Autodesk Inventor part; units mm, degrees
(part 2 of 2)
sketch "스케치10" plane through (0, 0, 4) normal (0, 0, 1) x (1, 0, 0)
  circle A0 centre (0, 0) radius 1.25 projected
  arc A1 (13.9479, -1.2066) -> (10.7334, 8.9886) centre (0, 0) ccw projected
  arc A2 (8.9665, -0.7757) -> (13.9479, -1.2066) centre (11.4572, -0.9911) ccw projected
  arc A3 (8.9665, -0.7757) -> (6.9, 5.7784) centre (0, 0) ccw projected
  arc A4 (10.7334, 8.9886) -> (6.9, 5.7784) centre (8.8167, 7.3835) ccw projected
  arc A5 (-8.0189, -11.476) -> (2.4176, -13.7897) centre (0, 0) ccw projected
  arc A6 (-5.155, -7.3774) -> (-8.0189, -11.476) centre (-6.5869, -9.4267) ccw projected
  arc A7 (-5.155, -7.3774) -> (1.5542, -8.8648) centre (0, 0) ccw projected
  arc A8 (2.4176, -13.7897) -> (1.5542, -8.8648) centre (1.9859, -11.3272) ccw projected
  arc A9 (-3.8115, 8.1531) -> (-8.4542, 3.0864) centre (0, 0) ccw projected
  arc A10 (-13.151, 4.8011) -> (-8.4542, 3.0864) centre (-10.8026, 3.9438) ccw projected
  arc A11 (-5.929, 12.6825) -> (-13.151, 4.8011) centre (0, 0) ccw projected
  arc A12 (-3.8115, 8.1531) -> (-5.929, 12.6825) centre (-4.8703, 10.4178) ccw projected
  circle A13 centre (-59.4867, -7.8316) radius 4.025 projected
  arc A14 (-60.1049, -2.02) -> (-65.4557, -8.4603) centre (-59.4744, -7.9868) ccw projected
  arc A15 (-65.4557, -8.4603) -> (-58.5717, -13.6038) centre (-59.507, -7.6772) ccw projected
  line L0 (-58.5717, -13.6038) -> (-20.5345, -7.6012) projected
  arc A16 (-19.9916, -7.9111) -> (-20.5345, -7.6012) centre (-20.4565, -8.0951) ccw projected
  arc A17 (-19.9916, -7.9111) -> (-19.7349, -8.5314) centre (0, 0) ccw projected
  arc A18 (-19.9027, -9.1363) -> (-19.7349, -8.5314) centre (-20.1938, -8.7298) ccw projected
  arc A19 (-19.9027, -9.1363) -> (-22.7962, -12.5032) centre (-14.4518, -16.7475) ccw projected
  arc A20 (-22.7962, -12.5032) -> (-22.2262, -13.4905) centre (0, 0) ccw projected
  arc A21 (-22.2262, -13.4905) -> (-17.8636, -12.6681) centre (-21.7297, -4.1418) ccw projected
  arc A22 (-17.2558, -12.8252) -> (-17.8636, -12.6681) centre (-17.6571, -13.1235) ccw projected
  arc A23 (-17.2558, -12.8252) -> (-16.8544, -13.3484) centre (0, 0) ccw projected
  arc A24 (-16.8599, -13.9762) -> (-16.8544, -13.3484) centre (-17.2463, -13.6589) ccw projected
  arc A25 (-16.8599, -13.9762) -> (-18.7834, -17.9773) centre (-9.6248, -19.9173) ccw projected
  arc A26 (-18.7834, -17.9773) -> (-17.9773, -18.7834) centre (0, 0) ccw projected
  arc A27 (-17.9773, -18.7834) -> (-13.9762, -16.8599) centre (-19.9173, -9.6248) ccw projected
  arc A28 (-13.3484, -16.8544) -> (-13.9762, -16.8599) centre (-13.6589, -17.2463) ccw projected
  arc A29 (-13.3484, -16.8544) -> (-12.8252, -17.2558) centre (0, 0) ccw projected
  arc A30 (-12.6681, -17.8636) -> (-12.8252, -17.2558) centre (-13.1235, -17.6571) ccw projected
  arc A31 (-12.6681, -17.8636) -> (-13.4905, -22.2262) centre (-4.1418, -21.7297) ccw projected
  arc A32 (-13.4905, -22.2262) -> (-12.5032, -22.7962) centre (0, 0) ccw projected
  arc A33 (-12.5032, -22.7962) -> (-9.1363, -19.9027) centre (-16.7475, -14.4518) ccw projected
  arc A34 (-8.5314, -19.7349) -> (-9.1363, -19.9027) centre (-8.7298, -20.1938) ccw projected
  arc A35 (-8.5314, -19.7349) -> (-7.9221, -19.9873) centre (0, 0) ccw projected
  arc A36 (-7.613, -20.5337) -> (-7.9221, -19.9873) centre (-8.1063, -20.4521) ccw projected
  arc A37 (-7.613, -20.5337) -> (-7.2783, -24.9605) centre (1.6233, -22.0613) ccw projected
  arc A38 (-7.2783, -24.9605) -> (-6.1771, -25.2556) centre (0, 0) ccw projected
  arc A39 (-6.1771, -25.2556) -> (-3.6738, -21.5892) centre (-12.4365, -18.2939) ccw projected
  arc A40 (-3.1329, -21.2705) -> (-3.6738, -21.5892) centre (-3.2058, -21.7652) ccw projected
  arc A41 (-3.1329, -21.2705) -> (-2.4791, -21.3566) centre (0, 0) ccw projected
  arc A42 (-2.0391, -21.8044) -> (-2.4791, -21.3566) centre (-2.5367, -21.8533) ccw projected
  arc A43 (-2.0391, -21.8044) -> (-0.57, -25.9938) centre (7.2779, -20.8894) ccw projected
  arc A44 (-0.57, -25.9938) -> (0.57, -25.9938) centre (0, 0) ccw projected
  arc A45 (0.57, -25.9938) -> (2.0391, -21.8044) centre (-7.2779, -20.8894) ccw projected
  arc A46 (2.4791, -21.3566) -> (2.0391, -21.8044) centre (2.5367, -21.8533) ccw projected
  arc A47 (2.4791, -21.3566) -> (3.1329, -21.2705) centre (0, 0) ccw projected
  arc A48 (3.6738, -21.5892) -> (3.1329, -21.2705) centre (3.2058, -21.7652) ccw projected
  arc A49 (3.6738, -21.5892) -> (6.1771, -25.2556) centre (12.4365, -18.2939) ccw projected
  arc A50 (6.1771, -25.2556) -> (7.2783, -24.9605) centre (0, 0) ccw projected
  arc A51 (7.2783, -24.9605) -> (7.613, -20.5337) centre (-1.6233, -22.0613) ccw projected
  arc A52 (7.9221, -19.9873) -> (7.613, -20.5337) centre (8.1063, -20.4521) ccw projected
  arc A53 (7.9221, -19.9873) -> (8.5314, -19.7349) centre (0, 0) ccw projected
  arc A54 (9.1363, -19.9027) -> (8.5314, -19.7349) centre (8.7298, -20.1938) ccw projected
  arc A55 (9.1363, -19.9027) -> (12.5032, -22.7962) centre (16.7475, -14.4518) ccw projected
  arc A56 (12.5032, -22.7962) -> (13.4905, -22.2262) centre (0, 0) ccw projected
  arc A57 (13.4905, -22.2262) -> (12.6681, -17.8636) centre (4.1418, -21.7297) ccw projected
  arc A58 (12.8252, -17.2558) -> (12.6681, -17.8636) centre (13.1235, -17.6571) ccw projected
  arc A59 (12.8252, -17.2558) -> (13.3484, -16.8544) centre (0, 0) ccw projected
  arc A60 (13.9762, -16.8599) -> (13.3484, -16.8544) centre (13.6589, -17.2463) ccw projected
  arc A61 (13.9762, -16.8599) -> (17.9773, -18.7834) centre (19.9173, -9.6248) ccw projected
  arc A62 (17.9773, -18.7834) -> (18.7834, -17.9773) centre (0, 0) ccw projected
  arc A63 (18.7834, -17.9773) -> (16.8599, -13.9762) centre (9.6248, -19.9173) ccw projected
  arc A64 (16.8544, -13.3484) -> (16.8599, -13.9762) centre (17.2463, -13.6589) ccw projected
  arc A65 (16.8544, -13.3484) -> (17.2558, -12.8252) centre (0, 0) ccw projected
  arc A66 (17.8636, -12.6681) -> (17.2558, -12.8252) centre (17.6571, -13.1235) ccw projected
  arc A67 (17.8636, -12.6681) -> (22.2262, -13.4905) centre (21.7297, -4.1418) ccw projected
  arc A68 (22.2262, -13.4905) -> (22.7962, -12.5032) centre (0, 0) ccw projected
  arc A69 (22.7962, -12.5032) -> (19.9027, -9.1363) centre (14.4518, -16.7475) ccw projected
  arc A70 (19.7349, -8.5314) -> (19.9027, -9.1363) centre (20.1938, -8.7298) ccw projected
  arc A71 (19.7349, -8.5314) -> (19.9873, -7.9221) centre (0, 0) ccw projected
  arc A72 (20.5337, -7.613) -> (19.9873, -7.9221) centre (20.4521, -8.1063) ccw projected
  arc A73 (20.5337, -7.613) -> (24.9605, -7.2783) centre (22.0613, 1.6233) ccw projected
  arc A74 (24.9605, -7.2783) -> (25.2556, -6.1771) centre (0, 0) ccw projected
  arc A75 (25.2556, -6.1771) -> (21.5892, -3.6738) centre (18.2939, -12.4365) ccw projected
  arc A76 (21.2705, -3.1329) -> (21.5892, -3.6738) centre (21.7652, -3.2058) ccw projected
  arc A77 (21.2705, -3.1329) -> (21.3566, -2.4791) centre (0, 0) ccw projected
  arc A78 (21.8044, -2.0391) -> (21.3566, -2.4791) centre (21.8533, -2.5367) ccw projected
  arc A79 (21.8044, -2.0391) -> (25.9938, -0.57) centre (20.8894, 7.2779) ccw projected
  arc A80 (25.9938, -0.57) -> (25.9938, 0.57) centre (0, 0) ccw projected
  arc A81 (25.9938, 0.57) -> (21.8044, 2.0391) centre (20.8894, -7.2779) ccw projected
  arc A82 (21.3566, 2.4791) -> (21.8044, 2.0391) centre (21.8533, 2.5367) ccw projected
  arc A83 (21.3566, 2.4791) -> (21.2705, 3.1329) centre (0, 0) ccw projected
  arc A84 (21.5892, 3.6738) -> (21.2705, 3.1329) centre (21.7652, 3.2058) ccw projected
  arc A85 (21.5892, 3.6738) -> (25.2556, 6.1771) centre (18.2939, 12.4365) ccw projected
  arc A86 (25.2556, 6.1771) -> (24.9605, 7.2783) centre (0, 0) ccw projected
  arc A87 (24.9605, 7.2783) -> (20.5337, 7.613) centre (22.0613, -1.6233) ccw projected
  arc A88 (19.9873, 7.9221) -> (20.5337, 7.613) centre (20.4521, 8.1063) ccw projected
  arc A89 (19.9873, 7.9221) -> (19.7349, 8.5314) centre (0, 0) ccw projected
  arc A90 (19.9027, 9.1363) -> (19.7349, 8.5314) centre (20.1938, 8.7298) ccw projected
  arc A91 (19.9027, 9.1363) -> (22.7962, 12.5032) centre (14.4518, 16.7475) ccw projected
  arc A92 (22.7962, 12.5032) -> (22.2262, 13.4905) centre (0, 0) ccw projected
  arc A93 (22.2262, 13.4905) -> (17.8636, 12.6681) centre (21.7297, 4.1418) ccw projected
  arc A94 (17.2558, 12.8252) -> (17.8636, 12.6681) centre (17.6571, 13.1235) ccw projected
  arc A95 (17.2558, 12.8252) -> (16.8544, 13.3484) centre (0, 0) ccw projected
  arc A96 (16.8599, 13.9762) -> (16.8544, 13.3484) centre (17.2463, 13.6589) ccw projected
  arc A97 (16.8599, 13.9762) -> (18.7834, 17.9773) centre (9.6248, 19.9173) ccw projected
  arc A98 (18.7834, 17.9773) -> (17.9773, 18.7834) centre (0, 0) ccw projected
  arc A99 (17.9773, 18.7834) -> (13.9762, 16.8599) centre (19.9173, 9.6248) ccw projected
  arc A100 (13.3484, 16.8544) -> (13.9762, 16.8599) centre (13.6589, 17.2463) ccw projected
  arc A101 (13.3484, 16.8544) -> (12.8252, 17.2558) centre (0, 0) ccw projected
  arc A102 (12.6681, 17.8636) -> (12.8252, 17.2558) centre (13.1235, 17.6571) ccw projected
  arc A103 (12.6681, 17.8636) -> (13.4905, 22.2262) centre (4.1418, 21.7297) ccw projected
  arc A104 (13.4905, 22.2262) -> (12.5032, 22.7962) centre (0, 0) ccw projected
  arc A105 (12.5032, 22.7962) -> (9.1363, 19.9027) centre (16.7475, 14.4518) ccw projected
  arc A106 (8.5314, 19.7349) -> (9.1363, 19.9027) centre (8.7298, 20.1938) ccw projected
  arc A107 (8.5314, 19.7349) -> (7.9221, 19.9873) centre (0, 0) ccw projected
  arc A108 (7.613, 20.5337) -> (7.9221, 19.9873) centre (8.1063, 20.4521) ccw projected
  arc A109 (7.613, 20.5337) -> (7.2783, 24.9605) centre (-1.6233, 22.0613) ccw projected
  arc A110 (7.2783, 24.9605) -> (6.1771, 25.2556) centre (0, 0) ccw projected
  arc A111 (6.1771, 25.2556) -> (3.6738, 21.5892) centre (12.4365, 18.2939) ccw projected
  arc A112 (3.1329, 21.2705) -> (3.6738, 21.5892) centre (3.2058, 21.7652) ccw projected
  arc A113 (3.1329, 21.2705) -> (2.4791, 21.3566) centre (0, 0) ccw projected
  arc A114 (2.0391, 21.8044) -> (2.4791, 21.3566) centre (2.5367, 21.8533) ccw projected
  arc A115 (2.0391, 21.8044) -> (0.57, 25.9938) centre (-7.2779, 20.8894) ccw projected
  arc A116 (0.57, 25.9938) -> (-0.57, 25.9938) centre (0, 0) ccw projected
  arc A117 (-0.57, 25.9938) -> (-2.0391, 21.8044) centre (7.2779, 20.8894) ccw projected
  arc A118 (-2.4791, 21.3566) -> (-2.0391, 21.8044) centre (-2.5367, 21.8533) ccw projected
  arc A119 (-2.4791, 21.3566) -> (-3.1329, 21.2705) centre (0, 0) ccw projected
  arc A120 (-3.6738, 21.5892) -> (-3.1329, 21.2705) centre (-3.2058, 21.7652) ccw projected
  arc A121 (-3.6738, 21.5892) -> (-6.1771, 25.2556) centre (-12.4365, 18.2939) ccw projected
  arc A122 (-6.1771, 25.2556) -> (-7.2783, 24.9605) centre (0, 0) ccw projected
  arc A123 (-7.2783, 24.9605) -> (-7.613, 20.5337) centre (1.6233, 22.0613) ccw projected
  arc A124 (-7.9221, 19.9873) -> (-7.613, 20.5337) centre (-8.1063, 20.4521) ccw projected
  arc A125 (-7.9221, 19.9873) -> (-8.5314, 19.7349) centre (0, 0) ccw projected
  arc A126 (-9.1363, 19.9027) -> (-8.5314, 19.7349) centre (-8.7298, 20.1938) ccw projected
  arc A127 (-9.1363, 19.9027) -> (-12.5032, 22.7962) centre (-16.7475, 14.4518) ccw projected
  arc A128 (-12.5032, 22.7962) -> (-13.4905, 22.2262) centre (0, 0) ccw projected
  arc A129 (-13.4905, 22.2262) -> (-12.6681, 17.8636) centre (-4.1418, 21.7297) ccw projected
  arc A130 (-12.8252, 17.2558) -> (-12.6681, 17.8636) centre (-13.1235, 17.6571) ccw projected
  arc A131 (-12.8252, 17.2558) -> (-13.3484, 16.8544) centre (0, 0) ccw projected
  arc A132 (-13.9762, 16.8599) -> (-13.3484, 16.8544) centre (-13.6589, 17.2463) ccw projected
  arc A133 (-13.9762, 16.8599) -> (-17.9773, 18.7834) centre (-19.9173, 9.6248) ccw projected
  arc A134 (-17.9773, 18.7834) -> (-18.7834, 17.9773) centre (0, 0) ccw projected
  arc A135 (-18.7834, 17.9773) -> (-16.8599, 13.9762) centre (-9.6248, 19.9173) ccw projected
  arc A136 (-16.8544, 13.3484) -> (-16.8599, 13.9762) centre (-17.2463, 13.6589) ccw projected
  arc A137 (-16.8544, 13.3484) -> (-17.2558, 12.8252) centre (0, 0) ccw projected
  arc A138 (-17.8636, 12.6681) -> (-17.2558, 12.8252) centre (-17.6571, 13.1235) ccw projected
  arc A139 (-17.8636, 12.6681) -> (-22.2262, 13.4905) centre (-21.7297, 4.1418) ccw projected
  arc A140 (-22.2262, 13.4905) -> (-22.7962, 12.5032) centre (0, 0) ccw projected
  arc A141 (-22.7962, 12.5032) -> (-19.9027, 9.1363) centre (-14.4518, 16.7475) ccw projected
  arc A142 (-19.7349, 8.5314) -> (-19.9027, 9.1363) centre (-20.1938, 8.7298) ccw projected
  arc A143 (-19.7349, 8.5314) -> (-19.9873, 7.9221) centre (0, 0) ccw projected
  arc A144 (-20.5337, 7.613) -> (-19.9873, 7.9221) centre (-20.4521, 8.1063) ccw projected
  arc A145 (-20.5337, 7.613) -> (-24.9605, 7.2783) centre (-22.0613, -1.6233) ccw projected
  arc A146 (-24.9605, 7.2783) -> (-25.2556, 6.1771) centre (0, 0) ccw projected
  arc A147 (-25.2556, 6.1771) -> (-21.5892, 3.6738) centre (-18.2939, 12.4365) ccw projected
  arc A148 (-21.2705, 3.1329) -> (-21.5892, 3.6738) centre (-21.7652, 3.2058) ccw projected
  arc A149 (-21.2705, 3.1329) -> (-21.358, 2.4674) centre (0, 0) ccw projected
  arc A150 (-21.8021, 2.0275) -> (-21.358, 2.4674) centre (-21.8546, 2.5248) ccw projected
  line L1 (-21.8021, 2.0275) -> (-60.1049, -2.02) projected
  circle A151 centre (0, 0) radius 1.25 projected
  circle A152 centre (0, 0) radius 1.6
  dimension "d53" = 3.2
  constraints: 1 centre point, 1 coincident
  measures "d53" diameter of A152
extrude "돌출10" cut sketch "스케치10" against normal blind 4 contours A152
